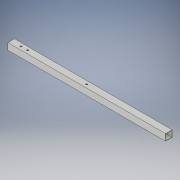
# Autodesk Inventor part: Short horizontal
Saved by Autodesk Inventor 2017 (Build 210142000, 142)
## iProperties
Created: 2018-07-12
Part Number: Short horizontal
Material: Generic
Document SubType Name: Modeling
Designer: sinner
Density: 1 g/cm^3
Appearance: Default
Author: sinner
Autodesk Inventor part; units mm, degrees
ref_plane "YZ Plane" through (0, 0, 0) normal (1, 0, 0) x (0, 1, 0)
ref_plane "XZ Plane" through (0, 0, 0) normal (0, 1, 0) x (-1, 0, 0)
ref_plane "XY Plane" through (0, 0, 0) normal (0, 0, 1) x (1, 0, 0)
sketch "Sketch1" plane through (0, 0, 0) normal (1, 0, 0) x (0, 1, 0)
  line L0 (0, 0) -> (25.4, 0)
  line L1 (25.4, 0) -> (25.4, -25.4)
  line L2 (25.4, -25.4) -> (0, -25.4)
  line L3 (0, -25.4) -> (0, 0)
  line L4 (23.8125, -1.5875) -> (1.5875, -1.5875)
  line L5 (1.5875, -1.5875) -> (1.5875, -23.8125)
  line L6 (1.5875, -23.8125) -> (23.8125, -23.8125)
  line L7 (23.8125, -23.8125) -> (23.8125, -1.5875)
  dimension "d0" = 25.4
  dimension "d1" = 25.4
  dimension "d2" = 1.5875
  constraints: 16 end point, 4 parallel, 2 perpendicular, 1 horizontal, 3 other
  measures "d0" distance of L1.end L2.end
  measures "d1" distance of L0.end L1.end
  measures "d2" distance between parallel lines of L1 L7
extrude "Extrusion1" add sketch "Sketch1" along normal blind 609.6
sketch "Sketch2" plane through (0, 25.4, 0) normal (0, 1, 0) x (1, 0, 0)
  line L0 (0, 1.5875) -> (0, 23.8125) projected
  line L1 (0, 12.7) -> (64.9449, 12.7) construction
  circle A0 centre (38.1, 12.7) radius 3.175
  circle A1 centre (63.5, 12.7) radius 3.175
  circle A2 centre (292.1, 12.7) radius 3.175
  point P0 (0, 0)
  dimension "d5" = 6.35
  dimension "d6" = 38.1
  dimension "d7" = 63.5
  dimension "d8" = 292.1
  constraints: 3 centre point, 3 point on line, 2 end point, 2 equal radius, 1 horizontal, 1 midpoint
  measures "d5" diameter of A0
  measures "d6" distance from line of L0 A0.centre
  measures "d7" distance from line of L0 A1.centre
  measures "d8" distance from line of L0 A2.centre
extrude "Extrusion2" cut sketch "Sketch2" against normal blind 25.4
body "Solid1"
